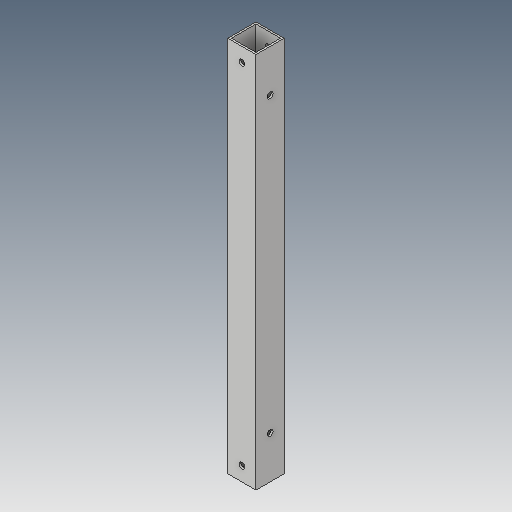
# Autodesk Inventor part: 回路角柱L200
Saved by Autodesk Inventor 2019.4 (Build 234330000, 330)
## iProperties
Created: 2018-06-23
Part Number: 回路角柱L200
Material: 一般
Document SubType Name: Modeling
Designer: AzLIer
Density: 1 g/cm^3
Appearance: 既定
Mass: 11.1357 g
Surface Area: 224.637 cm^2
Volume: 11.1357 cm^3
Author: AzLIer
Autodesk Inventor part; units mm, degrees
ref_plane "YZ Plane" through (0, 0, 0) normal (1, 0, 0) x (0, 1, 0)
ref_plane "XZ Plane" through (0, 0, 0) normal (0, 1, 0) x (-1, 0, 0)
ref_plane "XY Plane" through (0, 0, 0) normal (0, 0, 1) x (1, 0, 0)
sketch "スケッチ1" plane through (0, 0, 0) normal (0, 1, 0) x (-1, 0, 0)
  line L0 (-7.5, -7.5) -> (7.5, -7.5)
  line L1 (7.5, -7.5) -> (7.5, 7.5)
  line L2 (7.5, 7.5) -> (-7.5, 7.5)
  line L3 (-7.5, 7.5) -> (-7.5, -7.5)
  line L4 (-7.5, -7.5) -> (7.5, 7.5) construction
  line L5 (7.5, -7.5) -> (-7.5, 7.5) construction
  line L6 (6.5, 6.5) -> (6.5, -6.5)
  line L7 (6.5, -6.5) -> (-6.5, -6.5)
  line L8 (-6.5, -6.5) -> (-6.5, 6.5)
  line L9 (-6.5, 6.5) -> (6.5, 6.5)
  point P0 (0, 0)
  dimension "d0" = 15
  dimension "d1" = 15
  constraints: 20 end point, 2 midpoint, 2 parallel, 1 horizontal, 1 perpendicular
  measures "d0" distance of L2.end L1.end
  measures "d1" distance of L1.end L0.end
extrude "押し出し1" add sketch "スケッチ1" along normal mid plane 200
sketch "スケッチ3" plane through (-7.5, -100, 7.5) normal (-1, 0, 0) x (0, 0, 1)
  line L0 (-7.5, 177.5) -> (-7.5, 22.5)
  line L1 (0, 0) -> (-15, 0) projected
  point P0 (-7.5, 100)
  point P1 (-7.5, 100)
  dimension "d20" = 22.5
  constraints: 3 coincident, 2 end point, 1 midpoint, 1 vertical
  measures "d20" distance from line of point (-7.5, 22.5) L1
hole "穴1" at (-7.5, 77.5, 0) at (-7.5, -77.5, 0) direction (1, 0, 0) diameter 3.2 end through all
sketch "スケッチ4" plane through (7.5, 100, -7.5) normal (0, 0, -1) x (-1, 0, 0)
  line L0 (7.5, -7.5) -> (7.5, -192.5)
  line L1 (15, -200) -> (0, -200) projected
  point P0 (7.5, -100)
  point P1 (7.5, -100)
  dimension "d21" = 7.5
  constraints: 3 coincident, 2 end point, 1 midpoint, 1 vertical
  measures "d21" distance from line of L1 point (7.5, -192.5)
hole "穴2" at (0, 92.5, -7.5) at (0, -92.5, -7.5) direction (0, 0, 1) diameter 3.2 end through all
